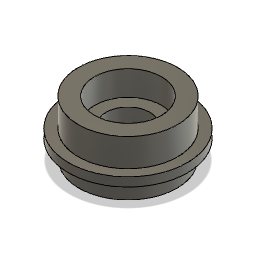
Injection mold holder _24well_cellvisplate (Autodesk Fusion 360 design; units mm, degrees)
Autodesk Fusion 360 part; units mm, degrees
sketch "Sketch1" plane through (0, 0, 0) normal (0, 1, 0) x (1, 0, 0)
  circle A0 centre (0, 0) radius 7.91
  circle A1 centre (0, 0) radius 3.5
  dimension "d1" = 15.82
  dimension "d2" = 7
  constraint coincident A0.centre A1.centre
  constraint concentric A0 A1
  measures "d1" diameter of A0
  measures "d2" diameter of A1
extrude "Extrude1" add sketch "Sketch1" along normal blind 3
sketch "Sketch2" plane through (0, 3, 0) normal (0, 1, 0) x (-1, 0, 0)
  circle A0 centre (0, 0) radius 3.5
  circle A1 centre (0, 0) radius 7.91
  circle A2 centre (0, 0) radius 9.6
  dimension "d5" = 19.2
  constraint concentric A0 A2
  measures "d5" diameter of A2
extrude "Extrude2" add sketch "Sketch2" along normal blind 6.932 contours A1 | A2
sketch "Sketch3" plane through (0, 9.932, 0) normal (0, 1, 0) x (-1, 0, 0)
  circle A0 centre (0, 0) radius 3.5
  circle A1 centre (0, 0) radius 9.6
  circle A2 centre (0, 0) radius 5.4
  dimension "d8" = 10.8
  constraint concentric A0 A2
  measures "d8" diameter of A2
extrude "Extrude3" cut sketch "Sketch3" against normal blind 3 contours A2
sketch "Sketch4" plane through (0, 9.932, 0) normal (0, 1, 0) x (-1, 0, 0)
  circle A0 centre (0, 0) radius 5.4
  circle A1 centre (0, 0) radius 9.6
  circle A2 centre (0, 0) radius 8
  constraint concentric A0 A2
extrude "Extrude4" cut sketch "Sketch4" against normal blind 5.5 contours A1
extrude "Extrude5" cut 1 faces at (-4.7335, 6.932, -0.4422) along direction (0, -1, 0) blind 2
extrude "Extrude6" cut 1 faces at (-7.0834, 9.932, -0.6657) along direction (0, -1, 0) blind 1
